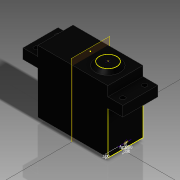
# Autodesk Inventor part: body
Saved by Autodesk Inventor 2013 (Build 170138000, 138)
## iProperties
Created: 2013-09-15
Part Number: body
Material: ABS Plastic
Document SubType Name: Modeling
Designer: Ian
Density: 1.06 g/cm^3
Mass: 33.708 g
Surface Area: 71.2072 cm^2
Volume: 31.8 cm^3
Author: Ian
Autodesk Inventor part; units mm, degrees
ref_plane "YZ Plane" through (0, 0, 0) normal (1, 0, 0) x (0, 1, 0)
ref_plane "XZ Plane" through (0, 0, 0) normal (0, 1, 0) x (-1, 0, 0)
ref_plane "XY Plane" through (0, 0, 0) normal (0, 0, 1) x (1, 0, 0)
sketch "Sketch1" plane through (0, 0, 0) normal (0, 1, 0) x (-1, 0, 0)
  line L0 (-20.2311, -10.16) -> (20.2311, -10.16)
  line L1 (20.2311, -10.16) -> (20.2311, 10.16)
  line L2 (20.2311, 10.16) -> (-20.2311, 10.16)
  line L3 (-20.2311, 10.16) -> (-20.2311, -10.16)
  line L4 (-20.2311, -10.16) -> (20.2311, 10.16) construction
  line L5 (20.2311, -10.16) -> (-20.2311, 10.16) construction
  point P0 (0, 0)
  dimension "d0" = 40.4622
  dimension "d1" = 20.32
  constraints: 12 end point, 2 midpoint, 2 parallel, 1 horizontal, 1 perpendicular
  measures "d0" distance of L2.end L1.end
  measures "d1" distance of L1.end L0.end
extrude "Extrusion1" add sketch "Sketch1" along normal blind 36.068
sketch "Sketch2" plane through (0, 36.068, 0) normal (0, 1, 0) x (1, 0, 0)
  line L0 (-20.2311, -10.16) -> (20.2311, -10.16) projected
  line L1 (20.2311, -10.16) -> (20.2311, 10.16) projected
  circle A0 centre (10.0711, 0) radius 6.985
  circle A1 centre (10.0711, 0) radius 5.08
  point P0 (0, 0)
  dimension "d4" = 13.97
  dimension "d5" = 10.16
  dimension "d6" = 10.16
  dimension "d7" = 10.16
  constraints: 2 centre point, 1 coincident
  measures "d4" diameter of A0
  measures "d5" distance from line of L1 A0.centre
  measures "d6" distance from line of L0 A0.centre
  measures "d7" diameter of A1
extrude "Extrusion2" add sketch "Sketch2" along normal blind 2.032 contours A1
chamfer "Chamfer1" distance 1.9812 angle 45 1 edges at (4.9911, 36.068, 0)
sketch "Sketch3" plane through (10.0711, 38.1, 0) normal (0, 1, 0) x (1, 0, 0)
  circle A0 centre (0, 0) radius 5.08 projected
  point P0 (-10.0711, 0)
  constraints: 1 coincident
ref_plane "Work Plane1" through (0, 38.1, 0) normal (1, 0, 0) x (0, 0, -1)
sketch "Sketch4" plane through (20.2311, 0, 10.16) normal (1, 0, 0) x (0, 0, -1)
  line L0 (20.32, 0) -> (20.32, 36.068) projected
  line L1 (0, 36.068) -> (20.32, 36.068)
  line L2 (20.32, 36.068) -> (20.32, 30.48)
  line L3 (20.32, 30.48) -> (0, 30.48)
  line L4 (0, 30.48) -> (0, 36.068)
  line L5 (0, 30.48) -> (20.32, 30.48)
  line L6 (20.32, 30.48) -> (20.32, 24.638)
  line L7 (20.32, 24.638) -> (0, 24.638)
  line L8 (0, 24.638) -> (0, 30.48)
  point P0 (10.16, 0)
  dimension "d14" = 5.588
  dimension "d16" = 5.842
  constraints: 16 end point, 4 parallel, 2 horizontal, 2 perpendicular, 2 point on line
  measures "d14" distance between parallel lines of L1 L3
  measures "d16" distance between parallel lines of L5 L7
extrude "Extrusion3" add sketch "Sketch4" along normal blind 8.636 contours L7 L8 L3 L0
sketch "Sketch5" plane through (20.2311, 30.48, 10.16) normal (0, 1, 0) x (1, 0, 0)
  line L0 (0, 0) -> (8.636, 0) projected
  line L1 (8.636, 20.32) -> (8.636, 0) projected
  line L2 (0, 20.32) -> (8.636, 20.32) projected
  point P0 (-20.2311, 10.16)
  point P1 (4.7752, 16.4592)
  point P2 (4.7752, 3.8608)
  dimension "d19" = 3.8608
  dimension "d20" = 3.8608
  dimension "d21" = 3.8608
  dimension "d22" = 3.8608
  measures "d19" distance from line of L2 point (4.775, 16.459)
  measures "d20" distance from line of L1 point (4.775, 16.459)
  measures "d21" distance from line of L1 point (4.775, 3.861)
  measures "d22" distance from line of L0 point (4.775, 3.861)
hole "Hole1" at (25.0063, 30.48, -6.2992) at (25.0063, 30.48, 6.2992) direction (0, -1, 0) diameter 2.7686 end through all
mirror "Mirror1" about plane through (0, 38.1, 0) normal (1, 0, 0) of "Extrusion3", "Hole1"
sketch "Sketch6" plane through (20.2311, 0, 10.16) normal (1, 0, 0) x (0, 0, -1)
  line L0 (20.32, 24.638) -> (0, 24.638) projected
  line L1 (0, 0) -> (0, 24.638) projected
  line L2 (0, 0) -> (20.32, 0) projected
  line L3 (20.32, 0) -> (20.32, 24.638) projected
  line L4 (5.7791, 2.54) -> (13.4355, 2.54)
  point P0 (10.16, 0)
  point P1 (10.16, 2.54)
  point P2 (10.922, 2.54)
  point P3 (9.398, 2.54)
  dimension "d30" = 0.762
  dimension "d32" = 0.762
  dimension "d33" = 0
  dimension "d34" = 2.54
  constraints: 3 point on line, 2 end point, 1 perpendicular
  measures "d30" distance of point (9.398, 2.54) point (10.16, 2.54)
  measures "d32" distance of point (10.922, 2.54) point (10.16, 2.54)
  measures "d33" horizontal distance of point (10.16, 2.54) point (10.16, 0)
  measures "d34" distance between parallel lines of L4 L2
equation "\"d32\" = d30"
body "Solid1"
